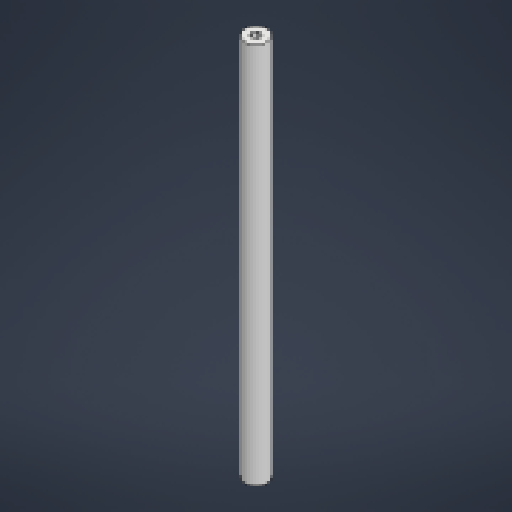
# Autodesk Inventor part: 3DPRINT,1.5inOD,DEAD-ROLLER
Saved by Autodesk Inventor 2026 (Build 300175000, 175)
## iProperties
Created: 2026-02-18
Part Number: 3DPRINT,1.5inOD,DEAD-ROLLER
Material: Generic
Document SubType Name: Modeling
Designer: littl
Density: 1 g/cm^3
Appearance: Default
Author: littl
Autodesk Inventor part; units mm, degrees
ref_plane "YZ Plane" through (0, 0, 0) normal (1, 0, 0) x (0, 1, 0)
ref_plane "XZ Plane" through (0, 0, 0) normal (0, 1, 0) x (-1, 0, 0)
ref_plane "XY Plane" through (0, 0, 0) normal (0, 0, 1) x (1, 0, 0)
sketch "Sketch1" plane through (0, 0, 0) normal (0, 1, 0) x (-1, 0, 0)
  circle A0 centre (0, 0) radius 19.05
  line L0 (-3.7395, -6.477) -> (-7.479, 0)
  line L1 (-7.479, 0) -> (-3.7395, 6.477)
  line L2 (-3.7395, 6.477) -> (3.7395, 6.477)
  line L3 (3.7395, 6.477) -> (7.479, 0)
  line L4 (7.479, 0) -> (3.7395, -6.477)
  line L5 (3.7395, -6.477) -> (-3.7395, -6.477)
  dimension "d0" = 38.1
  dimension "d1" = 12.954
  constraints: 12 end point, 2 coincident, 1 centre point, 1 horizontal, 13 other
  measures "d0" diameter of A0
  measures "d1" distance between parallel lines of L2 L5
extrude "Extrusion1" add sketch "Sketch1" along normal blind 647.7
body "Solid1"
